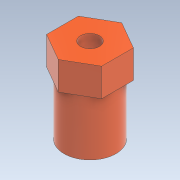
# Autodesk Inventor part: Coupling
Saved by Autodesk Inventor 2022 (Build 260153000, 153)
## iProperties
Created: 2023-03-17
Part Number: Coupling
Material: 一般
Document SubType Name: Modeling
Designer: JOU
Density: 1 g/cm^3
Appearance: 預設
Mass: 1.64153 g
Surface Area: 11.3377 cm^2
Volume: 1.64153 cm^3
Author: JOU
Autodesk Inventor part; units mm, degrees
ref_plane "XZ Plane" through (0, 0, 0) normal (0, 1, 0) x (-1, 0, 0)
ref_plane "XY Plane" through (0, 0, 0) normal (0, 0, 1) x (1, 0, 0)
sketch "草圖1" plane through (0, 0, 0) normal (0, 1, 0) x (-1, 0, 0)
  circle A0 centre (0, 0) radius 5.5
  dimension "d0" = 11
  constraints: 1 centre point, 1 coincident
  measures "d0" diameter of A0
extrude "擠出1" add sketch "草圖1" along normal blind 12
sketch "草圖2" plane through (0, 12, 0) normal (0, 1, 0) x (1, 0, 0)
  line L0 (5.85, -3.3775) -> (0, -6.755)
  line L1 (0, -6.755) -> (-5.85, -3.3775)
  line L2 (-5.85, -3.3775) -> (-5.85, 3.3775)
  line L3 (-5.85, 3.3775) -> (0, 6.755)
  line L4 (0, 6.755) -> (5.85, 3.3775)
  line L5 (5.85, 3.3775) -> (5.85, -3.3775)
  point P0 (0, 0)
  point P1 (0, 0)
  dimension "d3" = 11.7
  constraints: 12 end point, 1 coincident, 1 vertical, 13 other
  measures "d3" distance between parallel lines of L5 L2
extrude "擠出2" add sketch "草圖2" along normal blind 6
sketch "草圖3" plane through (0, 0, 0) normal (0, -1, 0) x (1, 0, 0)
  circle A0 centre (0, 0) radius 2
  dimension "d6" = 4
  constraints: 1 centre point, 1 coincident
  measures "d6" diameter of A0
extrude "擠出3" cut sketch "草圖3" against normal up to surface (18 mm away)
sketch "草圖6" plane through (0, 0, 0) normal (0, -1, 0) x (1, 0, 0)
  circle A0 centre (0, 0) radius 2 projected
  circle A1 centre (0, 0) radius 5.5 projected
  circle A2 centre (0, 0) radius 2 projected
  line L0 (1.0536, 1.7) -> (-1.0536, 1.7)
  dimension "d15" = 1.7
  constraints: 2 end point, 2 point on circle, 1 horizontal
  measures "d15" distance from line of L0 point (0, 0)
ref_plane "工作平面2" through (-5.5, 0, 0) normal (1, 0, 0) x (0, 1, 0)
ref_plane "工作平面1" through (5.5, 0, 0) normal (1, 0, 0) x (0, 1, 0)
sketch "草圖8" plane through (0, 0, 0) normal (0, -1, 0) x (1, 0, 0)
  arc A0 (-0.7518, 6.0636) -> (-1.1588, 5.9991) centre (0, 0) ccw
  arc A1 (-1.1588, 5.9991) -> (-1.2788, 5.8304) centre (-1.1303, 5.8518) ccw
  arc A2 (-1.2782, 5.5484) -> (-1.2788, 5.8304) centre (-2.2685, 5.6874) ccw
  arc A3 (-2.2271, 5.24) -> (-1.2782, 5.5484) centre (-1.8278, 5.6255) ccw
  arc A4 (-2.3924, 5.4685) -> (-2.2271, 5.24) centre (-1.5077, 5.9346) ccw
  arc A5 (-2.3924, 5.4685) -> (-2.5887, 5.5345) centre (-2.5252, 5.3986) ccw
  arc A6 (-2.5887, 5.5345) -> (-2.9559, 5.3474) centre (0, 0) ccw
  arc A7 (-2.9559, 5.3474) -> (-3.0179, 5.1498) centre (-2.8833, 5.2161) ccw
  arc A8 (-2.9302, 4.8818) -> (-3.0179, 5.1498) centre (-3.915, 4.708) ccw
  arc A9 (-3.7374, 4.2953) -> (-2.9302, 4.8818) centre (-3.4767, 4.7853) ccw
  arc A10 (-3.9652, 4.4616) -> (-3.7374, 4.2953) centre (-3.2678, 5.1782) ccw
  arc A11 (-3.9652, 4.4616) -> (-4.1723, 4.4637) centre (-4.0698, 4.3541) ccw
  arc A12 (-4.1723, 4.4637) -> (-4.4637, 4.1723) centre (0, 0) ccw
  arc A13 (-4.4637, 4.1723) -> (-4.4616, 3.9652) centre (-4.3541, 4.0698) ccw
  arc A14 (-4.2953, 3.7374) -> (-4.4616, 3.9652) centre (-5.1782, 3.2678) ccw
  arc A15 (-4.8818, 2.9302) -> (-4.2953, 3.7374) centre (-4.7853, 3.4767) ccw
  arc A16 (-5.1498, 3.0179) -> (-4.8818, 2.9302) centre (-4.708, 3.915) ccw
  arc A17 (-5.1498, 3.0179) -> (-5.3474, 2.9559) centre (-5.2161, 2.8833) ccw
  arc A18 (-5.3474, 2.9559) -> (-5.5345, 2.5887) centre (0, 0) ccw
  arc A19 (-5.5345, 2.5887) -> (-5.4685, 2.3924) centre (-5.3986, 2.5252) ccw
  arc A20 (-5.24, 2.2271) -> (-5.4685, 2.3924) centre (-5.9346, 1.5077) ccw
  arc A21 (-5.5484, 1.2782) -> (-5.24, 2.2271) centre (-5.6255, 1.8278) ccw
  arc A22 (-5.8304, 1.2788) -> (-5.5484, 1.2782) centre (-5.6874, 2.2685) ccw
  arc A23 (-5.8304, 1.2788) -> (-5.9991, 1.1588) centre (-5.8518, 1.1303) ccw
  arc A24 (-5.9991, 1.1588) -> (-6.0636, 0.7518) centre (0, 0) ccw
  arc A25 (-6.0636, 0.7518) -> (-5.9402, 0.5855) centre (-5.9147, 0.7333) ccw
  arc A26 (-5.6718, 0.4989) -> (-5.9402, 0.5855) centre (-6.11, -0.4) ccw
  arc A27 (-5.6718, -0.4989) -> (-5.6718, 0.4989) centre (-5.915, 0) ccw
  arc A28 (-5.9402, -0.5855) -> (-5.6718, -0.4989) centre (-6.11, 0.4) ccw
  arc A29 (-5.9402, -0.5855) -> (-6.0636, -0.7518) centre (-5.9147, -0.7333) ccw
  arc A30 (-6.0636, -0.7518) -> (-5.9991, -1.1588) centre (0, 0) ccw
  arc A31 (-5.9991, -1.1588) -> (-5.8304, -1.2788) centre (-5.8518, -1.1303) ccw
  arc A32 (-5.5484, -1.2782) -> (-5.8304, -1.2788) centre (-5.6874, -2.2685) ccw
  arc A33 (-5.24, -2.2271) -> (-5.5484, -1.2782) centre (-5.6255, -1.8278) ccw
  arc A34 (-5.4685, -2.3924) -> (-5.24, -2.2271) centre (-5.9346, -1.5077) ccw
  arc A35 (-5.4685, -2.3924) -> (-5.5345, -2.5887) centre (-5.3986, -2.5252) ccw
  arc A36 (-5.5345, -2.5887) -> (-5.3474, -2.9559) centre (0, 0) ccw
  arc A37 (-5.3474, -2.9559) -> (-5.1498, -3.0179) centre (-5.2161, -2.8833) ccw
  arc A38 (-4.8818, -2.9302) -> (-5.1498, -3.0179) centre (-4.708, -3.915) ccw
  arc A39 (-4.2953, -3.7374) -> (-4.8818, -2.9302) centre (-4.7853, -3.4767) ccw
  arc A40 (-4.4616, -3.9652) -> (-4.2953, -3.7374) centre (-5.1782, -3.2678) ccw
  arc A41 (-4.4616, -3.9652) -> (-4.4637, -4.1723) centre (-4.3541, -4.0698) ccw
  arc A42 (-4.4637, -4.1723) -> (-4.1723, -4.4637) centre (0, 0) ccw
  arc A43 (-4.1723, -4.4637) -> (-3.9652, -4.4616) centre (-4.0698, -4.3541) ccw
  arc A44 (-3.7374, -4.2953) -> (-3.9652, -4.4616) centre (-3.2678, -5.1782) ccw
  arc A45 (-2.9302, -4.8818) -> (-3.7374, -4.2953) centre (-3.4767, -4.7853) ccw
  arc A46 (-3.0179, -5.1498) -> (-2.9302, -4.8818) centre (-3.915, -4.708) ccw
  arc A47 (-3.0179, -5.1498) -> (-2.9559, -5.3474) centre (-2.8833, -5.2161) ccw
  arc A48 (-2.9559, -5.3474) -> (-2.5887, -5.5345) centre (0, 0) ccw
  arc A49 (-2.5887, -5.5345) -> (-2.3924, -5.4685) centre (-2.5252, -5.3986) ccw
  arc A50 (-2.2271, -5.24) -> (-2.3924, -5.4685) centre (-1.5077, -5.9346) ccw
  arc A51 (-1.2782, -5.5484) -> (-2.2271, -5.24) centre (-1.8278, -5.6255) ccw
  arc A52 (-1.2788, -5.8304) -> (-1.2782, -5.5484) centre (-2.2685, -5.6874) ccw
  arc A53 (-1.2788, -5.8304) -> (-1.1588, -5.9991) centre (-1.1303, -5.8518) ccw
  arc A54 (-1.1588, -5.9991) -> (-0.7518, -6.0636) centre (0, 0) ccw
  arc A55 (-0.7518, -6.0636) -> (-0.5855, -5.9402) centre (-0.7333, -5.9147) ccw
  arc A56 (-0.4989, -5.6718) -> (-0.5855, -5.9402) centre (0.4, -6.11) ccw
  arc A57 (0.4989, -5.6718) -> (-0.4989, -5.6718) centre (0, -5.915) ccw
  arc A58 (0.5855, -5.9402) -> (0.4989, -5.6718) centre (-0.4, -6.11) ccw
  arc A59 (0.5855, -5.9402) -> (0.7518, -6.0636) centre (0.7333, -5.9147) ccw
  arc A60 (0.7518, -6.0636) -> (1.1588, -5.9991) centre (0, 0) ccw
  arc A61 (1.1588, -5.9991) -> (1.2788, -5.8304) centre (1.1303, -5.8518) ccw
  arc A62 (1.2782, -5.5484) -> (1.2788, -5.8304) centre (2.2685, -5.6874) ccw
  arc A63 (2.2271, -5.24) -> (1.2782, -5.5484) centre (1.8278, -5.6255) ccw
  arc A64 (2.3924, -5.4685) -> (2.2271, -5.24) centre (1.5077, -5.9346) ccw
  arc A65 (2.3924, -5.4685) -> (2.5887, -5.5345) centre (2.5252, -5.3986) ccw
  arc A66 (2.5887, -5.5345) -> (2.9559, -5.3474) centre (0, 0) ccw
  arc A67 (2.9559, -5.3474) -> (3.0179, -5.1498) centre (2.8833, -5.2161) ccw
  arc A68 (2.9302, -4.8818) -> (3.0179, -5.1498) centre (3.915, -4.708) ccw
  arc A69 (3.7374, -4.2953) -> (2.9302, -4.8818) centre (3.4767, -4.7853) ccw
  arc A70 (3.9652, -4.4616) -> (3.7374, -4.2953) centre (3.2678, -5.1782) ccw
  arc A71 (3.9652, -4.4616) -> (4.1723, -4.4637) centre (4.0698, -4.3541) ccw
  arc A72 (4.1723, -4.4637) -> (4.4637, -4.1723) centre (0, 0) ccw
  arc A73 (4.4637, -4.1723) -> (4.4616, -3.9652) centre (4.3541, -4.0698) ccw
  arc A74 (4.2953, -3.7374) -> (4.4616, -3.9652) centre (5.1782, -3.2678) ccw
  arc A75 (4.8818, -2.9302) -> (4.2953, -3.7374) centre (4.7853, -3.4767) ccw
  arc A76 (5.1498, -3.0179) -> (4.8818, -2.9302) centre (4.708, -3.915) ccw
  arc A77 (5.1498, -3.0179) -> (5.3474, -2.9559) centre (5.2161, -2.8833) ccw
  arc A78 (5.3474, -2.9559) -> (5.5345, -2.5887) centre (0, 0) ccw
  arc A79 (5.5345, -2.5887) -> (5.4685, -2.3924) centre (5.3986, -2.5252) ccw
  arc A80 (5.24, -2.2271) -> (5.4685, -2.3924) centre (5.9346, -1.5077) ccw
  arc A81 (5.5484, -1.2782) -> (5.24, -2.2271) centre (5.6255, -1.8278) ccw
  arc A82 (5.8304, -1.2788) -> (5.5484, -1.2782) centre (5.6874, -2.2685) ccw
  arc A83 (5.8304, -1.2788) -> (5.9991, -1.1588) centre (5.8518, -1.1303) ccw
  arc A84 (5.9991, -1.1588) -> (6.0636, -0.7518) centre (0, 0) ccw
  arc A85 (6.0636, -0.7518) -> (5.9402, -0.5855) centre (5.9147, -0.7333) ccw
  arc A86 (5.6718, -0.4989) -> (5.9402, -0.5855) centre (6.11, 0.4) ccw
  arc A87 (5.6718, 0.4989) -> (5.6718, -0.4989) centre (5.915, 0) ccw
  arc A88 (5.9402, 0.5855) -> (5.6718, 0.4989) centre (6.11, -0.4) ccw
  arc A89 (5.9402, 0.5855) -> (6.0636, 0.7518) centre (5.9147, 0.7333) ccw
  arc A90 (6.0636, 0.7518) -> (5.9991, 1.1588) centre (0, 0) ccw
  arc A91 (5.9991, 1.1588) -> (5.8304, 1.2788) centre (5.8518, 1.1303) ccw
  arc A92 (5.5484, 1.2782) -> (5.8304, 1.2788) centre (5.6874, 2.2685) ccw
  arc A93 (5.24, 2.2271) -> (5.5484, 1.2782) centre (5.6255, 1.8278) ccw
  arc A94 (5.4685, 2.3924) -> (5.24, 2.2271) centre (5.9346, 1.5077) ccw
  arc A95 (5.4685, 2.3924) -> (5.5345, 2.5887) centre (5.3986, 2.5252) ccw
  arc A96 (5.5345, 2.5887) -> (5.3474, 2.9559) centre (0, 0) ccw
  arc A97 (5.3474, 2.9559) -> (5.1498, 3.0179) centre (5.2161, 2.8833) ccw
  arc A98 (4.8818, 2.9302) -> (5.1498, 3.0179) centre (4.708, 3.915) ccw
  arc A99 (4.2953, 3.7374) -> (4.8818, 2.9302) centre (4.7853, 3.4767) ccw
  arc A100 (4.4616, 3.9652) -> (4.2953, 3.7374) centre (5.1782, 3.2678) ccw
  arc A101 (4.4616, 3.9652) -> (4.4637, 4.1723) centre (4.3541, 4.0698) ccw
  arc A102 (4.4637, 4.1723) -> (4.1723, 4.4637) centre (0, 0) ccw
  arc A103 (4.1723, 4.4637) -> (3.9652, 4.4616) centre (4.0698, 4.3541) ccw
  arc A104 (3.7374, 4.2953) -> (3.9652, 4.4616) centre (3.2678, 5.1782) ccw
  arc A105 (2.9302, 4.8818) -> (3.7374, 4.2953) centre (3.4767, 4.7853) ccw
  arc A106 (3.0179, 5.1498) -> (2.9302, 4.8818) centre (3.915, 4.708) ccw
  arc A107 (3.0179, 5.1498) -> (2.9559, 5.3474) centre (2.8833, 5.2161) ccw
  arc A108 (2.9559, 5.3474) -> (2.5887, 5.5345) centre (0, 0) ccw
  arc A109 (2.5887, 5.5345) -> (2.3924, 5.4685) centre (2.5252, 5.3986) ccw
  arc A110 (2.2271, 5.24) -> (2.3924, 5.4685) centre (1.5077, 5.9346) ccw
  arc A111 (1.2782, 5.5484) -> (2.2271, 5.24) centre (1.8278, 5.6255) ccw
  arc A112 (1.2788, 5.8304) -> (1.2782, 5.5484) centre (2.2685, 5.6874) ccw
  arc A113 (1.2788, 5.8304) -> (1.1588, 5.9991) centre (1.1303, 5.8518) ccw
  arc A114 (1.1588, 5.9991) -> (0.7518, 6.0636) centre (0, 0) ccw
  arc A115 (0.7518, 6.0636) -> (0.5855, 5.9402) centre (0.7333, 5.9147) ccw
  arc A116 (0.4989, 5.6718) -> (0.5855, 5.9402) centre (-0.4, 6.11) ccw
  arc A117 (-0.4989, 5.6718) -> (0.4989, 5.6718) centre (0, 5.915) ccw
  arc A118 (-0.5855, 5.9402) -> (-0.4989, 5.6718) centre (0.4, 6.11) ccw
  arc A119 (-0.5855, 5.9402) -> (-0.7518, 6.0636) centre (-0.7333, 5.9147) ccw
  constraints: 240 point on circle, 120 centre point
extrude "擠出7" [suppressed]
sketch "草圖9" plane through (0, 0, 0) normal (0, 1, 0) x (1, 0, 0)
  point P0 (0, 0)
extrude "擠出8" [suppressed]
sketch "草圖10" plane through (0, 0, 0) normal (0, -1, 0) x (1, 0, 0)
  arc A0 (-5.5, 0) -> (-5.5, 0) centre (0, 0) ccw projected
  arc A1 (-5.5, 0) -> (-5.5, 0) centre (0, 0) ccw projected
  circle A2 centre (0, 0) radius 5.5 projected
  arc A3 (-0.7518, 6.0636) -> (-1.1588, 5.9991) centre (0, 0) ccw projected
  arc A4 (-1.1588, 5.9991) -> (-1.2788, 5.8304) centre (-1.1303, 5.8518) ccw projected
  arc A5 (-1.2782, 5.5484) -> (-1.2788, 5.8304) centre (-2.2685, 5.6874) ccw projected
  arc A6 (-2.2271, 5.24) -> (-1.2782, 5.5484) centre (-1.8278, 5.6255) ccw projected
  arc A7 (-2.3924, 5.4685) -> (-2.2271, 5.24) centre (-1.5077, 5.9346) ccw projected
  arc A8 (-2.3924, 5.4685) -> (-2.5887, 5.5345) centre (-2.5252, 5.3986) ccw projected
  arc A9 (-2.5887, 5.5345) -> (-2.9559, 5.3474) centre (0, 0) ccw projected
  arc A10 (-2.9559, 5.3474) -> (-3.0179, 5.1498) centre (-2.8833, 5.2161) ccw projected
  arc A11 (-2.9302, 4.8818) -> (-3.0179, 5.1498) centre (-3.915, 4.708) ccw projected
  arc A12 (-3.7374, 4.2953) -> (-2.9302, 4.8818) centre (-3.4767, 4.7853) ccw projected
  arc A13 (-3.9652, 4.4616) -> (-3.7374, 4.2953) centre (-3.2678, 5.1782) ccw projected
  arc A14 (-3.9652, 4.4616) -> (-4.1723, 4.4637) centre (-4.0698, 4.3541) ccw projected
  arc A15 (-4.1723, 4.4637) -> (-4.4637, 4.1723) centre (0, 0) ccw projected
  arc A16 (-4.4637, 4.1723) -> (-4.4616, 3.9652) centre (-4.3541, 4.0698) ccw projected
  arc A17 (-4.2953, 3.7374) -> (-4.4616, 3.9652) centre (-5.1782, 3.2678) ccw projected
  arc A18 (-4.8818, 2.9302) -> (-4.2953, 3.7374) centre (-4.7853, 3.4767) ccw projected
  arc A19 (-5.1498, 3.0179) -> (-4.8818, 2.9302) centre (-4.708, 3.915) ccw projected
  arc A20 (-5.1498, 3.0179) -> (-5.3474, 2.9559) centre (-5.2161, 2.8833) ccw projected
  arc A21 (-5.3474, 2.9559) -> (-5.5345, 2.5887) centre (0, 0) ccw projected
  arc A22 (-5.5345, 2.5887) -> (-5.4685, 2.3924) centre (-5.3986, 2.5252) ccw projected
  arc A23 (-5.24, 2.2271) -> (-5.4685, 2.3924) centre (-5.9346, 1.5077) ccw projected
  arc A24 (-5.5484, 1.2782) -> (-5.24, 2.2271) centre (-5.6255, 1.8278) ccw projected
  arc A25 (-5.8304, 1.2788) -> (-5.5484, 1.2782) centre (-5.6874, 2.2685) ccw projected
  arc A26 (-5.8304, 1.2788) -> (-5.9991, 1.1588) centre (-5.8518, 1.1303) ccw projected
  arc A27 (-5.9991, 1.1588) -> (-6.0636, 0.7518) centre (0, 0) ccw projected
  arc A28 (-6.0636, 0.7518) -> (-5.9402, 0.5855) centre (-5.9147, 0.7333) ccw projected
  arc A29 (-5.6718, 0.4989) -> (-5.9402, 0.5855) centre (-6.11, -0.4) ccw projected
  arc A30 (-5.6718, -0.4989) -> (-5.6718, 0.4989) centre (-5.915, 0) ccw projected
  arc A31 (-5.9402, -0.5855) -> (-5.6718, -0.4989) centre (-6.11, 0.4) ccw projected
  arc A32 (-5.9402, -0.5855) -> (-6.0636, -0.7518) centre (-5.9147, -0.7333) ccw projected
  arc A33 (-6.0636, -0.7518) -> (-5.9991, -1.1588) centre (0, 0) ccw projected
  arc A34 (-5.9991, -1.1588) -> (-5.8304, -1.2788) centre (-5.8518, -1.1303) ccw projected
  arc A35 (-5.5484, -1.2782) -> (-5.8304, -1.2788) centre (-5.6874, -2.2685) ccw projected
  arc A36 (-5.24, -2.2271) -> (-5.5484, -1.2782) centre (-5.6255, -1.8278) ccw projected
  arc A37 (-5.4685, -2.3924) -> (-5.24, -2.2271) centre (-5.9346, -1.5077) ccw projected
  arc A38 (-5.4685, -2.3924) -> (-5.5345, -2.5887) centre (-5.3986, -2.5252) ccw projected
  arc A39 (-5.5345, -2.5887) -> (-5.3474, -2.9559) centre (0, 0) ccw projected
  arc A40 (-5.3474, -2.9559) -> (-5.1498, -3.0179) centre (-5.2161, -2.8833) ccw projected
  arc A41 (-4.8818, -2.9302) -> (-5.1498, -3.0179) centre (-4.708, -3.915) ccw projected
  arc A42 (-4.2953, -3.7374) -> (-4.8818, -2.9302) centre (-4.7853, -3.4767) ccw projected
  arc A43 (-4.4616, -3.9652) -> (-4.2953, -3.7374) centre (-5.1782, -3.2678) ccw projected
  arc A44 (-4.4616, -3.9652) -> (-4.4637, -4.1723) centre (-4.3541, -4.0698) ccw projected
  arc A45 (-4.4637, -4.1723) -> (-4.1723, -4.4637) centre (0, 0) ccw projected
  arc A46 (-4.1723, -4.4637) -> (-3.9652, -4.4616) centre (-4.0698, -4.3541) ccw projected
  arc A47 (-3.7374, -4.2953) -> (-3.9652, -4.4616) centre (-3.2678, -5.1782) ccw projected
  arc A48 (-2.9302, -4.8818) -> (-3.7374, -4.2953) centre (-3.4767, -4.7853) ccw projected
  arc A49 (-3.0179, -5.1498) -> (-2.9302, -4.8818) centre (-3.915, -4.708) ccw projected
  arc A50 (-3.0179, -5.1498) -> (-2.9559, -5.3474) centre (-2.8833, -5.2161) ccw projected
  arc A51 (-2.9559, -5.3474) -> (-2.5887, -5.5345) centre (0, 0) ccw projected
  arc A52 (-2.5887, -5.5345) -> (-2.3924, -5.4685) centre (-2.5252, -5.3986) ccw projected
  arc A53 (-2.2271, -5.24) -> (-2.3924, -5.4685) centre (-1.5077, -5.9346) ccw projected
  arc A54 (-1.2782, -5.5484) -> (-2.2271, -5.24) centre (-1.8278, -5.6255) ccw projected
  arc A55 (-1.2788, -5.8304) -> (-1.2782, -5.5484) centre (-2.2685, -5.6874) ccw projected
  arc A56 (-1.2788, -5.8304) -> (-1.1588, -5.9991) centre (-1.1303, -5.8518) ccw projected
  arc A57 (-1.1588, -5.9991) -> (-0.7518, -6.0636) centre (0, 0) ccw projected
  arc A58 (-0.7518, -6.0636) -> (-0.5855, -5.9402) centre (-0.7333, -5.9147) ccw projected
  arc A59 (-0.4989, -5.6718) -> (-0.5855, -5.9402) centre (0.4, -6.11) ccw projected
  arc A60 (0.4989, -5.6718) -> (-0.4989, -5.6718) centre (0, -5.915) ccw projected
  arc A61 (0.5855, -5.9402) -> (0.4989, -5.6718) centre (-0.4, -6.11) ccw projected
  arc A62 (0.5855, -5.9402) -> (0.7518, -6.0636) centre (0.7333, -5.9147) ccw projected
  arc A63 (0.7518, -6.0636) -> (1.1588, -5.9991) centre (0, 0) ccw projected
  arc A64 (1.1588, -5.9991) -> (1.2788, -5.8304) centre (1.1303, -5.8518) ccw projected
  arc A65 (1.2782, -5.5484) -> (1.2788, -5.8304) centre (2.2685, -5.6874) ccw projected
  arc A66 (2.2271, -5.24) -> (1.2782, -5.5484) centre (1.8278, -5.6255) ccw projected
  arc A67 (2.3924, -5.4685) -> (2.2271, -5.24) centre (1.5077, -5.9346) ccw projected
  arc A68 (2.3924, -5.4685) -> (2.5887, -5.5345) centre (2.5252, -5.3986) ccw projected
  arc A69 (2.5887, -5.5345) -> (2.9559, -5.3474) centre (0, 0) ccw projected
  arc A70 (2.9559, -5.3474) -> (3.0179, -5.1498) centre (2.8833, -5.2161) ccw projected
  arc A71 (2.9302, -4.8818) -> (3.0179, -5.1498) centre (3.915, -4.708) ccw projected
  arc A72 (3.7374, -4.2953) -> (2.9302, -4.8818) centre (3.4767, -4.7853) ccw projected
  arc A73 (3.9652, -4.4616) -> (3.7374, -4.2953) centre (3.2678, -5.1782) ccw projected
  arc A74 (3.9652, -4.4616) -> (4.1723, -4.4637) centre (4.0698, -4.3541) ccw projected
  arc A75 (4.1723, -4.4637) -> (4.4637, -4.1723) centre (0, 0) ccw projected
  arc A76 (4.4637, -4.1723) -> (4.4616, -3.9652) centre (4.3541, -4.0698) ccw projected
  arc A77 (4.2953, -3.7374) -> (4.4616, -3.9652) centre (5.1782, -3.2678) ccw projected
  arc A78 (4.8818, -2.9302) -> (4.2953, -3.7374) centre (4.7853, -3.4767) ccw projected
  arc A79 (5.1498, -3.0179) -> (4.8818, -2.9302) centre (4.708, -3.915) ccw projected
  arc A80 (5.1498, -3.0179) -> (5.3474, -2.9559) centre (5.2161, -2.8833) ccw projected
  arc A81 (5.3474, -2.9559) -> (5.5345, -2.5887) centre (0, 0) ccw projected
  arc A82 (5.5345, -2.5887) -> (5.4685, -2.3924) centre (5.3986, -2.5252) ccw projected
  arc A83 (5.24, -2.2271) -> (5.4685, -2.3924) centre (5.9346, -1.5077) ccw projected
  arc A84 (5.5484, -1.2782) -> (5.24, -2.2271) centre (5.6255, -1.8278) ccw projected
  arc A85 (5.8304, -1.2788) -> (5.5484, -1.2782) centre (5.6874, -2.2685) ccw projected
  arc A86 (5.8304, -1.2788) -> (5.9991, -1.1588) centre (5.8518, -1.1303) ccw projected
  arc A87 (5.9991, -1.1588) -> (6.0636, -0.7518) centre (0, 0) ccw projected
  arc A88 (6.0636, -0.7518) -> (5.9402, -0.5855) centre (5.9147, -0.7333) ccw projected
  arc A89 (5.6718, -0.4989) -> (5.9402, -0.5855) centre (6.11, 0.4) ccw projected
  arc A90 (5.6718, 0.4989) -> (5.6718, -0.4989) centre (5.915, 0) ccw projected
  arc A91 (5.9402, 0.5855) -> (5.6718, 0.4989) centre (6.11, -0.4) ccw projected
  arc A92 (5.9402, 0.5855) -> (6.0636, 0.7518) centre (5.9147, 0.7333) ccw projected
  arc A93 (6.0636, 0.7518) -> (5.9991, 1.1588) centre (0, 0) ccw projected
  arc A94 (5.9991, 1.1588) -> (5.8304, 1.2788) centre (5.8518, 1.1303) ccw projected
  arc A95 (5.5484, 1.2782) -> (5.8304, 1.2788) centre (5.6874, 2.2685) ccw projected
  arc A96 (5.24, 2.2271) -> (5.5484, 1.2782) centre (5.6255, 1.8278) ccw projected
  arc A97 (5.4685, 2.3924) -> (5.24, 2.2271) centre (5.9346, 1.5077) ccw projected
  arc A98 (5.4685, 2.3924) -> (5.5345, 2.5887) centre (5.3986, 2.5252) ccw projected
  arc A99 (5.5345, 2.5887) -> (5.3474, 2.9559) centre (0, 0) ccw projected
  arc A100 (5.3474, 2.9559) -> (5.1498, 3.0179) centre (5.2161, 2.8833) ccw projected
  arc A101 (4.8818, 2.9302) -> (5.1498, 3.0179) centre (4.708, 3.915) ccw projected
  arc A102 (4.2953, 3.7374) -> (4.8818, 2.9302) centre (4.7853, 3.4767) ccw projected
  arc A103 (4.4616, 3.9652) -> (4.2953, 3.7374) centre (5.1782, 3.2678) ccw projected
  arc A104 (4.4616, 3.9652) -> (4.4637, 4.1723) centre (4.3541, 4.0698) ccw projected
  arc A105 (4.4637, 4.1723) -> (4.1723, 4.4637) centre (0, 0) ccw projected
  arc A106 (4.1723, 4.4637) -> (3.9652, 4.4616) centre (4.0698, 4.3541) ccw projected
  arc A107 (3.7374, 4.2953) -> (3.9652, 4.4616) centre (3.2678, 5.1782) ccw projected
  arc A108 (2.9302, 4.8818) -> (3.7374, 4.2953) centre (3.4767, 4.7853) ccw projected
  arc A109 (3.0179, 5.1498) -> (2.9302, 4.8818) centre (3.915, 4.708) ccw projected
  arc A110 (3.0179, 5.1498) -> (2.9559, 5.3474) centre (2.8833, 5.2161) ccw projected
  arc A111 (2.9559, 5.3474) -> (2.5887, 5.5345) centre (0, 0) ccw projected
  arc A112 (2.5887, 5.5345) -> (2.3924, 5.4685) centre (2.5252, 5.3986) ccw projected
  arc A113 (2.2271, 5.24) -> (2.3924, 5.4685) centre (1.5077, 5.9346) ccw projected
  arc A114 (1.2782, 5.5484) -> (2.2271, 5.24) centre (1.8278, 5.6255) ccw projected
  arc A115 (1.2788, 5.8304) -> (1.2782, 5.5484) centre (2.2685, 5.6874) ccw projected
  arc A116 (1.2788, 5.8304) -> (1.1588, 5.9991) centre (1.1303, 5.8518) ccw projected
  arc A117 (1.1588, 5.9991) -> (0.7518, 6.0636) centre (0, 0) ccw projected
  arc A118 (0.7518, 6.0636) -> (0.5855, 5.9402) centre (0.7333, 5.9147) ccw projected
  arc A119 (0.4989, 5.6718) -> (0.5855, 5.9402) centre (-0.4, 6.11) ccw projected
  arc A120 (-0.4989, 5.6718) -> (0.4989, 5.6718) centre (0, 5.915) ccw projected
  arc A121 (-0.5855, 5.9402) -> (-0.4989, 5.6718) centre (0.4, 6.11) ccw projected
  arc A122 (-0.5855, 5.9402) -> (-0.7518, 6.0636) centre (-0.7333, 5.9147) ccw projected
  point P0 (4.6491, -2.9387)
  point P1 (4.2315, -3.5134)
  point P2 (1.3583, 5.3296)
  point P3 (2.0338, 5.1101)
  point P4 (-5.4885, -0.3552)
  point P5 (-5.4885, 0.3552)
  point P6 (-2.0338, 5.1101)
  point P7 (-1.3583, 5.3296)
  point P8 (2.9387, 4.6491)
  point P9 (3.5134, 4.2315)
  point P10 (5.1101, 2.0338)
  point P11 (5.3296, 1.3583)
  point P12 (5.3296, -1.3583)
  point P13 (5.1101, -2.0338)
  point P14 (2.0338, -5.1101)
  point P15 (1.3583, -5.3296)
  point P16 (-2.9387, -4.6491)
  point P17 (-3.5134, -4.2315)
  point P18 (-5.1101, -2.0338)
  point P19 (-5.3296, -1.3583)
  point P20 (-4.6491, 2.9387)
  point P21 (-4.2315, 3.5134)
  point P22 (0.3552, -5.4885)
  point P23 (-0.3552, -5.4885)
  point P24 (-0.3552, 5.4885)
  point P25 (0.3552, 5.4885)
  point P26 (4.2315, 3.5134)
  point P27 (4.6491, 2.9387)
  point P28 (5.4885, 0.3552)
  point P29 (5.4885, -0.3552)
  point P30 (3.5134, -4.2315)
  point P31 (2.9387, -4.6491)
  point P32 (-1.3583, -5.3296)
  point P33 (-2.0338, -5.1101)
  point P34 (-4.2315, -3.5134)
  point P35 (-4.6491, -2.9387)
  point P36 (-5.3296, 1.3583)
  point P37 (-5.1101, 2.0338)
  point P38 (-3.5134, 4.2315)
  point P39 (-2.9387, 4.6491)
  point P40 (0.3552, 5.4885)
  point P41 (-0.3552, 5.4885)
  point P42 (0.3552, 5.4885)
  point P43 (-0.3552, 5.4885)
  constraints: 1 other
extrude "擠出9" [suppressed]
sketch "草圖11" plane through (0, 1, 0) normal (0, 1, 0) x (1, 0, 0)
  circle A0 centre (0, 0) radius 5.5 projected
  circle A1 centre (0, 0) radius 6.5
  arc A2 (-4.2315, 3.5134) -> (-4.6491, 2.9387) centre (0, 0) ccw projected
  point P0 (5.4885, -0.3552)
  point P1 (5.4885, 0.3552)
  dimension "d26" = 13
  constraints: 1 centre point, 1 concentric
  measures "d26" diameter of A1
extrude "擠出10" [suppressed]
sketch "草圖5" plane through (0, 0, 0) normal (1, 0, 0) x (0, 1, 0)
  circle A0 centre (-2, 0) radius 1.475
  line L0 (0, 21.2872) -> (0, -21.2872) projected
  line L1 (1, -6.5) -> (1, 6.5) projected
  point P0 (0, 0)
  dimension "d32" = 3
  dimension "d33" = 2.95
  constraints: 1 centre point, 1 horizontal alignment
  measures "d32" distance from line of A0.centre L1
  measures "d33" diameter of A0
extrude "擠出5" [suppressed]
sketch "草圖7" plane through (-5.5, 0, 0) normal (1, 0, 0) x (0, 1, 0)
  circle A0 centre (-2, 0) radius 1.525
  point P0 (0, 0)
  point P1 (-2, 0)
  dimension "d17" = 3.05
  constraints: 1 centre point, 1 coincident
  measures "d17" diameter of A0
extrude "擠出6" [suppressed]
mirror "鏡射1" [suppressed]
sketch "草圖12" plane through (0, 18, 0) normal (0, 1, 0) x (1, 0, 0)
  circle A0 centre (0, 0) radius 2 projected
extrude "擠出11" [suppressed]
sketch "草圖13" plane through (0, -5, 0) normal (0, -1, 0) x (1, 0, 0)
  circle A0 centre (0, 0) radius 2.125
  dimension "d38" = 4.25
  constraints: 1 centre point, 1 coincident
  measures "d38" diameter of A0
extrude "擠出12" [suppressed]
